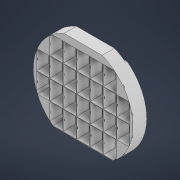
# Autodesk Inventor part: LuggageHoneyComb
Saved by Autodesk Inventor 2021 (Build 250183000, 183)
## iProperties
Created: 2021-01-31
Part Number: LuggageHoneyComb
Material: Generic
Document SubType Name: Modeling
Designer: argon
Density: 1 g/cm^3
Appearance: Default
Author: argon
Autodesk Inventor part; units mm, degrees
ref_plane "YZ Plane" through (0, 0, 0) normal (1, 0, 0) x (0, 1, 0)
ref_plane "XZ Plane" through (0, 0, 0) normal (0, 1, 0) x (-1, 0, 0)
ref_plane "XY Plane" through (0, 0, 0) normal (0, 0, 1) x (1, 0, 0)
sketch "Sketch1" plane through (0, 0, 0) normal (0, 0, 1) x (1, 0, 0)
  circle A0 centre (0, 0) radius 1740
  line L0 (-1391.658, -1044.4559) -> (-1392.1676, 1043.7765)
  circle A1 centre (0, 0) radius 1750
  line L1 (-1050, -1400) -> (1050, -1400)
  line L2 (245, -1400) -> (-245, -1400)
  line L3 (-245, -1400) -> (-245, -688)
  line L4 (-245, -688) -> (245, -688)
  line L5 (245, -688) -> (245, -1400)
  line L6 (-225, -708) -> (225, -708)
  line L7 (225, -708) -> (225, -1380)
  line L8 (225, -1380) -> (-225, -1380)
  line L9 (-225, -1380) -> (-225, -708)
  line L10 (245, -708) -> (695, -708)
  line L11 (225, -688) -> (715, -688)
  line L12 (715, -688) -> (715, -1400)
  line L13 (695, -708) -> (695, -1380)
  line L14 (245, -1380) -> (245, -708)
  line L15 (225, -1400) -> (225, -688)
  line L16 (695, -1380) -> (245, -1380)
  line L17 (715, -1400) -> (225, -1400)
  line L18 (715, -708) -> (1165, -708)
  line L19 (695, -688) -> (1185, -688)
  line L20 (1185, -688) -> (1185, -1400)
  line L21 (1165, -708) -> (1165, -1380)
  line L22 (715, -1380) -> (715, -708)
  line L23 (695, -1400) -> (695, -688)
  line L24 (1165, -1380) -> (715, -1380)
  line L25 (1185, -1400) -> (695, -1400)
  line L26 (1185, -708) -> (1635, -708)
  line L27 (1165, -688) -> (1655, -688)
  line L28 (1655, -688) -> (1655, -1400)
  line L29 (1635, -708) -> (1635, -1380)
  line L30 (1185, -1380) -> (1185, -708)
  line L31 (1165, -1400) -> (1165, -688)
  line L32 (1635, -1380) -> (1185, -1380)
  line L33 (1655, -1400) -> (1165, -1400)
  line L34 (-715, -688) -> (-225, -688)
  line L35 (-695, -708) -> (-245, -708)
  line L36 (-715, -1400) -> (-715, -688)
  line L37 (-695, -1380) -> (-695, -708)
  line L38 (-225, -688) -> (-225, -1400)
  line L39 (-245, -1400) -> (-245, -688)
  line L40 (-245, -1380) -> (-695, -1380)
  line L41 (-225, -1400) -> (-715, -1400)
  line L42 (-225, -1380) -> (-225, -708)
  line L43 (-1185, -688) -> (-695, -688)
  line L44 (-1165, -708) -> (-715, -708)
  line L45 (-1185, -1400) -> (-1185, -688)
  line L46 (-1165, -1380) -> (-1165, -708)
  line L47 (-695, -688) -> (-695, -1400)
  line L48 (-715, -1400) -> (-715, -688)
  line L49 (-715, -1380) -> (-1165, -1380)
  line L50 (-695, -1400) -> (-1185, -1400)
  line L51 (-695, -1380) -> (-695, -708)
  line L52 (-1655, -688) -> (-1165, -688)
  line L53 (-1635, -708) -> (-1185, -708)
  line L54 (-1655, -1400) -> (-1655, -688)
  line L55 (-1635, -1380) -> (-1635, -708)
  line L56 (-1165, -688) -> (-1165, -1400)
  line L57 (-1185, -1400) -> (-1185, -688)
  line L58 (-1185, -1380) -> (-1635, -1380)
  line L59 (-1165, -1400) -> (-1655, -1400)
  line L60 (-1165, -1380) -> (-1165, -708)
  line L61 (225, -688) -> (-225, -688)
  line L62 (245, -708) -> (-245, -708)
  line L63 (-225, -688) -> (-225, -16)
  line L64 (-225, 4) -> (-225, -708)
  line L65 (-245, -708) -> (-245, 4)
  line L66 (-245, -708) -> (-245, 4)
  line L67 (-695, -16) -> (-245, -16)
  line L68 (-715, 4) -> (-225, 4)
  line L69 (-245, -688) -> (-695, -688)
  line L70 (-225, -708) -> (-715, -708)
  line L71 (-225, -688) -> (-225, -16)
  line L72 (-695, 4) -> (-695, -708)
  line L73 (-715, -708) -> (-715, 4)
  line L74 (-695, -688) -> (-695, -16)
  line L75 (695, -16) -> (695, -688)
  line L76 (715, -688) -> (715, -16)
  line L77 (695, -708) -> (695, 4)
  line L78 (715, 4) -> (715, -708)
  line L79 (715, -16) -> (1165, -16)
  line L80 (1165, -688) -> (715, -688)
  line L81 (1165, -708) -> (1165, 4)
  line L82 (1185, -708) -> (695, -708)
  line L83 (695, 4) -> (1185, 4)
  line L84 (695, -688) -> (245, -688)
  line L85 (245, 4) -> (245, -708)
  line L86 (245, -688) -> (245, -16)
  line L87 (715, -708) -> (225, -708)
  line L88 (225, -708) -> (225, 4)
  line L89 (225, -16) -> (225, -688)
  line L90 (245, -16) -> (695, -16)
  line L91 (225, 4) -> (715, 4)
  line L92 (-245, 4) -> (245, 4)
  line L93 (-225, -16) -> (225, -16)
  line L94 (-715, -708) -> (-715, 4)
  line L95 (-695, -688) -> (-695, -16)
  line L96 (-1165, 4) -> (-1165, -708)
  line L97 (-715, -688) -> (-1165, -688)
  line L98 (-1165, -688) -> (-1165, -16)
  line L99 (-695, -708) -> (-1185, -708)
  line L100 (-1185, -708) -> (-1185, 4)
  line L101 (-1165, -16) -> (-715, -16)
  line L102 (-1185, 4) -> (-695, 4)
  line L103 (-1185, -708) -> (-1185, 4)
  line L104 (-1165, -688) -> (-1165, -16)
  line L105 (-1635, -16) -> (-1185, -16)
  line L106 (-1635, -688) -> (-1635, -16)
  line L107 (-1655, 4) -> (-1165, 4)
  line L108 (-1655, -708) -> (-1655, 4)
  line L109 (-1185, -688) -> (-1635, -688)
  line L110 (-1165, -708) -> (-1655, -708)
  line L111 (1185, 4) -> (1185, -708)
  line L112 (1165, -16) -> (1165, -688)
  line L113 (1185, -688) -> (1185, -16)
  line L114 (1635, -16) -> (1635, -688)
  line L115 (1635, -688) -> (1185, -688)
  line L116 (1655, 4) -> (1655, -708)
  line L117 (1655, -708) -> (1165, -708)
  line L118 (1185, -16) -> (1635, -16)
  line L119 (1165, 4) -> (1655, 4)
  line L120 (225, 4) -> (-225, 4)
  line L121 (245, -16) -> (-245, -16)
  line L122 (-225, 4) -> (-225, 676)
  line L123 (-225, 696) -> (-225, -16)
  line L124 (-245, -16) -> (-245, 696)
  line L125 (-245, -16) -> (-245, 696)
  line L126 (-695, 676) -> (-245, 676)
  line L127 (-715, 696) -> (-225, 696)
  line L128 (-245, 4) -> (-695, 4)
  line L129 (-225, -16) -> (-715, -16)
  line L130 (-225, 4) -> (-225, 676)
  line L131 (-695, 696) -> (-695, -16)
  line L132 (-715, -16) -> (-715, 696)
  line L133 (-695, 4) -> (-695, 676)
  line L134 (695, 676) -> (695, 4)
  line L135 (715, 4) -> (715, 676)
  line L136 (695, -16) -> (695, 696)
  line L137 (715, 696) -> (715, -16)
  line L138 (715, 676) -> (1165, 676)
  line L139 (1165, 4) -> (715, 4)
  line L140 (1165, -16) -> (1165, 696)
  line L141 (1185, -16) -> (695, -16)
  line L142 (695, 696) -> (1185, 696)
  line L143 (695, 4) -> (245, 4)
  line L144 (245, 696) -> (245, -16)
  line L145 (245, 4) -> (245, 676)
  line L146 (715, -16) -> (225, -16)
  line L147 (225, -16) -> (225, 696)
  line L148 (225, 676) -> (225, 4)
  line L149 (245, 676) -> (695, 676)
  line L150 (225, 696) -> (715, 696)
  line L151 (-245, 696) -> (245, 696)
  line L152 (-225, 676) -> (225, 676)
  line L153 (-715, -16) -> (-715, 696)
  line L154 (-695, 4) -> (-695, 676)
  line L155 (-1165, 696) -> (-1165, -16)
  line L156 (-715, 4) -> (-1165, 4)
  line L157 (-1165, 4) -> (-1165, 676)
  line L158 (-695, -16) -> (-1185, -16)
  line L159 (-1185, -16) -> (-1185, 696)
  line L160 (-1165, 676) -> (-715, 676)
  line L161 (-1185, 696) -> (-695, 696)
  line L162 (-1185, -16) -> (-1185, 696)
  line L163 (-1165, 4) -> (-1165, 676)
  line L164 (-1635, 676) -> (-1185, 676)
  line L165 (-1635, 4) -> (-1635, 676)
  line L166 (-1655, 696) -> (-1165, 696)
  line L167 (-1655, -16) -> (-1655, 696)
  line L168 (-1185, 4) -> (-1635, 4)
  line L169 (-1165, -16) -> (-1655, -16)
  line L170 (1185, 696) -> (1185, -16)
  line L171 (1165, 676) -> (1165, 4)
  line L172 (1185, 4) -> (1185, 676)
  line L173 (1635, 676) -> (1635, 4)
  line L174 (1635, 4) -> (1185, 4)
  line L175 (1655, 696) -> (1655, -16)
  line L176 (1655, -16) -> (1165, -16)
  line L177 (1185, 676) -> (1635, 676)
  line L178 (1165, 696) -> (1655, 696)
  line L179 (225, 696) -> (-225, 696)
  line L180 (245, 676) -> (-245, 676)
  line L181 (-225, 696) -> (-225, 1368)
  line L182 (-225, 1388) -> (-225, 676)
  line L183 (-245, 676) -> (-245, 1388)
  line L184 (-245, 676) -> (-245, 1388)
  line L185 (-695, 1368) -> (-245, 1368)
  line L186 (-715, 1388) -> (-225, 1388)
  line L187 (-245, 696) -> (-695, 696)
  line L188 (-225, 676) -> (-715, 676)
  line L189 (-225, 696) -> (-225, 1368)
  line L190 (-695, 1388) -> (-695, 676)
  line L191 (-715, 676) -> (-715, 1388)
  line L192 (-695, 696) -> (-695, 1368)
  line L193 (695, 1368) -> (695, 696)
  line L194 (715, 696) -> (715, 1368)
  line L195 (695, 676) -> (695, 1388)
  line L196 (715, 1388) -> (715, 676)
  line L197 (715, 1368) -> (1165, 1368)
  line L198 (1165, 696) -> (715, 696)
  line L199 (1165, 676) -> (1165, 1388)
  line L200 (1185, 676) -> (695, 676)
  line L201 (695, 1388) -> (1185, 1388)
  line L202 (695, 696) -> (245, 696)
  line L203 (245, 1388) -> (245, 676)
  line L204 (245, 696) -> (245, 1368)
  line L205 (715, 676) -> (225, 676)
  line L206 (225, 676) -> (225, 1388)
  line L207 (225, 1368) -> (225, 696)
  line L208 (245, 1368) -> (695, 1368)
  line L209 (225, 1388) -> (715, 1388)
  line L210 (-245, 1388) -> (245, 1388)
  line L211 (-225, 1368) -> (225, 1368)
  line L212 (-715, 676) -> (-715, 1388)
  line L213 (-695, 696) -> (-695, 1368)
  line L214 (-1165, 1388) -> (-1165, 676)
  line L215 (-715, 696) -> (-1165, 696)
  line L216 (-1165, 696) -> (-1165, 1368)
  line L217 (-695, 676) -> (-1185, 676)
  line L218 (-1185, 676) -> (-1185, 1388)
  line L219 (-1165, 1368) -> (-715, 1368)
  line L220 (-1185, 1388) -> (-695, 1388)
  line L221 (-1185, 676) -> (-1185, 1388)
  line L222 (-1165, 696) -> (-1165, 1368)
  line L223 (-1635, 1368) -> (-1185, 1368)
  line L224 (-1635, 696) -> (-1635, 1368)
  line L225 (-1655, 1388) -> (-1165, 1388)
  line L226 (-1655, 676) -> (-1655, 1388)
  line L227 (-1185, 696) -> (-1635, 696)
  line L228 (-1165, 676) -> (-1655, 676)
  line L229 (1185, 1388) -> (1185, 676)
  line L230 (1165, 1368) -> (1165, 696)
  line L231 (1185, 696) -> (1185, 1368)
  line L232 (1635, 1368) -> (1635, 696)
  line L233 (1635, 696) -> (1185, 696)
  line L234 (1655, 1388) -> (1655, 676)
  line L235 (1655, 676) -> (1165, 676)
  line L236 (1185, 1368) -> (1635, 1368)
  line L237 (1165, 1388) -> (1655, 1388)
  line L238 (-666.7653, 1618) -> (666.7653, 1618)
  point P0 (0, -708)
  point P1 (470, -708)
  point P2 (940, -708)
  point P3 (1410, -708)
  point P4 (-470, -708)
  point P5 (-940, -708)
  point P6 (-1410, -708)
  point P7 (1050, -708)
  point P8 (-470, -16)
  point P9 (-1050, -708)
  point P10 (940, -16)
  point P11 (470, -16)
  point P12 (0, -16)
  point P13 (-940, -16)
  point P14 (-1410, -16)
  point P15 (1410, -16)
  point P16 (1050, -16)
  point P17 (-470, 676)
  point P18 (-1050, -16)
  point P19 (940, 676)
  point P20 (470, 676)
  point P21 (0, 676)
  point P22 (-940, 676)
  point P23 (-1410, 676)
  point P24 (1410, 676)
  point P25 (1050, 676)
  point P26 (-470, 1368)
  point P27 (-1050, 676)
  point P28 (940, 1368)
  point P29 (470, 1368)
  point P30 (0, 1368)
  point P31 (-940, 1368)
  point P32 (-1410, 1368)
  point P33 (1410, 1368)
  point P34 (1059.8113, -1380)
  point P35 (1165, -1292.4299)
  point P36 (245, -1380)
  point P37 (1598.204, -688)
  point P38 (1635, -595.294)
  point P39 (-695, -16)
  point P40 (1165, -16)
  point P41 (245, 4)
  point P42 (225, 1368)
  point P43 (245, 696)
  point P44 (1075.2562, 1368)
  point P45 (1165, 1292.4299)
  point P46 (-1165, 1292.4299)
  point P47 (-1075.2562, 1368)
  point P48 (-715, 1368)
  point P49 (1603.3166, 676)
  point P50 (1635, 595.294)
  point P51 (-1635, 595.294)
  point P52 (-1603.3166, 676)
  point P53 (-245, 1368)
  point P54 (1165, 676)
  point P55 (245, -688)
  point P56 (-1598.204, -688)
  point P57 (-1635, -595.294)
  point P58 (-1059.8113, -1380)
  point P59 (-1165, -1292.4299)
  point P60 (-245, -1380)
  point P61 (-245, -708)
  point P62 (1065.8124, 1388)
  point P63 (-1065.8124, 1388)
  dimension "d7" = 1400
  dimension "d8" = 3500
  dimension "d9" = 490
  dimension "d10" = 712
  dimension "d11" = 20
  dimension "d12" = 20
  dimension "d13" = 20
  dimension "d14" = 20
  dimension "d17" = 470
  dimension "d24" = 470
  dimension "d31" = 692
  dimension "d36" = 10
  dimension "d41" = 230
  constraints: 478 end point, 6 horizontal, 6 point on circle, 4 parallel, 2 centre point, 2 perpendicular, 1 coincident, 1 collinear, 1 midpoint, 1 point on line, 1 vertical, 1 vertical alignment, 525 other
  measures "d7" distance from line of L1 A0.centre
  measures "d8" diameter of A1
  measures "d9" distance of L3.end L4.end
  measures "d10" distance of L4.end L2.start
  measures "d11" distance between parallel lines of L7 L5
  measures "d12" distance between parallel lines of L4 L6
  measures "d13" distance between parallel lines of L3 L9
  measures "d14" distance between parallel lines of L2 L8
  measures "d17" distance of L6.start L10.start
  measures "d24" distance of L3.end L34.start
  measures "d31" distance of L1.end point (1050, -708)
  measures "d36" radial gap between concentric circles of A0 A1
  measures "d41" distance between parallel lines of L210 L238
extrude "Extrusion1" add sketch "Sketch1" along normal blind 431.8 contours A0 L116 L175 | A0 L175 A1 L116 | L175 L119 L173 A0 | A0 L173 A1 L175 | L116 A1 L114 A0 | A0 L114 L176 L116 | A0 L177 A1 L173 | L116 L176 L118 L111 L119 | L114 A1 L27 A0 | L177 L170 L178 A0 | A0 L178 A1 L177 | L27 A1 L26 A0 | A0 L26 L20 L27 | L178 L229 A0 | A0 L229 A1 L178 | L200 L140 L142 L170 | L170 L83 L140 L200 | L111 L141 L81 L83 | L26 A1 L20 A0 | A0 L20 L26 | L20 L82 L31 L19 | L19 L81 L141 L111 | L229 L142 L199 A0 | A0 L199 A1 L229 | L138 L137 L142 L140 | L81 L79 L78 L83 | L20 A1 L21 A0 | A0 L21 L82 L20 | L31 L18 L12 L19 | A0 L197 A1 L199 | L200 L136 L142 L137 | L135 L83 L134 L200 | L78 L141 L77 L83 | L21 A1 L24 A0 | L12 L82 L23 L11 | L11 L75 L141 L76 | L197 L196 L201 A0 | A0 L201 A1 L197 | L142 L193 L195 L201 L196 L194 | L149 L144 L150 L136 | L77 L90 L85 L91 | L24 A1 L1 A0 | A0 L1 L12 L24 | L12 L1 L23 L13 L82 | L23 L10 L5 L11 | L201 L209 L210 L186 L220 A0 L238 | A0 L238 A1 L201 | L180 L147 L150 L144 | L144 L91 L147 L180 | L85 L121 L88 L91 | L5 L62 L15 L4 | L4 L88 L121 L85 | L150 L206 L209 L203 | L208 L203 L209 L195 | L152 L123 L151 L147 | L88 L93 L64 L92 | L1 A1 L49 A0 | A0 L49 L36 L1 | L5 L1 L15 L7 L62 | L23 L1 L5 L16 | L15 L6 L38 L4 | A0 L220 A1 L238 | L180 L124 L127 L123 | L122 L68 L124 L180 | L64 L121 L65 L68 | L49 A1 L46 A0 | L36 L70 L37 L47 L1 | L38 L62 L3 L4 | L4 L65 L121 L63 | L220 L191 L219 A0 | A0 L219 A1 L220 | L127 L183 L186 L182 L181 | L211 L182 L210 L206 | L126 L131 L127 L124 | L65 L67 L72 L68 | L46 A1 L45 A0 | A0 L45 L99 L46 | L47 L40 L3 L1 | L9 L38 L1 L3 L62 | L15 L1 L38 L8 | L3 L35 L47 L34 | A0 L214 A1 L219 | L186 L190 L127 L191 | L188 L132 L127 L131 | L131 L68 L132 L188 | L72 L129 L73 L68 | L45 A1 L53 A0 | A0 L0 L53 L45 | L56 L43 L36 L44 | L99 L45 L43 L56 | L36 L34 L47 L70 | L34 L73 L129 L72 | L214 L161 L218 A0 | A0 L218 A1 L214 | L186 L183 L185 L190 | L160 L155 L161 L132 | L73 L101 L96 L102 | A0 L53 L0 | L53 L0 L52 L45 | L43 L100 L158 L96 | A1 L52 A0 L53 | L218 L166 L0 A0 | A0 L166 A1 L218 | L155 L217 L159 L161 | L155 L102 L159 L217 | L96 L158 L100 L102 | A0 L52 L0 L53 | A1 L106 A0 L52 | L0 L166 A0 | L159 L164 L0 L166 | L100 L105 L0 L107 | L166 A0 L164 A1 | A1 L108 A0 L106 | A1 L167 A0 L108 | L166 L0 L164 A0 | L0 L105 L169 L108 L107 | L164 A0 L165 A1 | A0 L108 L169 L106 | A1 L165 A0 L167 | A0 L167 L108 | L107 L167 A0 L165
sketch "Sketch2" plane through (0, 0, 0) normal (0, 0, -1) x (-1, 0, 0)
  circle A0 centre (0, 0) radius 1750
  arc A1 (-666.7653, 1618) -> (-1050, -1400) centre (0, 0) ccw projected
  line L0 (-1065.8124, 1388) -> (1065.8124, 1388) projected
  line L1 (1065.8124, 1388) -> (-1065.8124, 1388)
  line L2 (1050, -1400) -> (-1050, -1400) projected
  line L3 (-1050, -1400) -> (1050, -1400)
  constraints: 4 end point, 1 centre point, 1 coincident, 1 collinear, 1 concentric, 1 horizontal
extrude "Extrusion2" add sketch "Sketch2" along normal blind 50 contours A0 L2 L0
sketch "Sketch5" plane through (225, 696, 431.8) normal (-1, 0, 0) x (0, 0, 1)
  line L0 (-30, 372) -> (-25, 372)
  line L1 (-25, 372) -> (-25, 300)
  line L2 (-25, 300) -> (-30, 300)
  line L3 (-30, 300) -> (-30, 372)
  line L4 (-30, -1012) -> (-25, -1012)
  line L5 (-25, -1012) -> (-25, -1084)
  line L6 (-25, -1084) -> (-30, -1084)
  line L7 (-30, -1084) -> (-30, -1012)
  line L8 (-25, -320) -> (-30, -320)
  line L9 (-30, -320) -> (-30, -392)
  line L10 (-30, -392) -> (-25, -392)
  line L11 (-25, -392) -> (-25, -320)
  line L12 (-30, -1704) -> (-35, -1704)
  line L13 (-35, -1704) -> (-35, -1776)
  line L14 (-35, -1776) -> (-30, -1776)
  line L15 (-30, -1776) -> (-30, -1704)
  line L16 (-431.8, -2076) -> (0, -2076) projected
  line L17 (0, -1404) -> (0, -2076) projected
  line L18 (-431.8, 0) -> (0, 0) projected
  line L19 (-431.8, -692) -> (0, -692) projected
  line L20 (-431.8, -1384) -> (0, -1384) projected
  point P0 (-431.8, -696)
  dimension "d42" = 72
  dimension "d43" = 5
  dimension "d44" = 300
  dimension "d45" = 30
  dimension "d46" = 300
  dimension "d47" = 300
  dimension "d48" = 300
  constraints: 32 end point, 14 parallel, 5 point on line, 4 horizontal, 4 perpendicular
  measures "d42" distance of L14.end L12.start
  measures "d43" distance of L12.start L12.end
  measures "d44" distance between parallel lines of L16 L14
  measures "d45" distance between parallel lines of L17 L15
  measures "d46" distance from line of L18 L1.end
  measures "d47" distance from line of L19 L10.end
  measures "d48" distance from line of L20 L5.end
extrude "Extrusion3" cut sketch "Sketch5" along normal through all both and the other way through all
body "Solid1"
